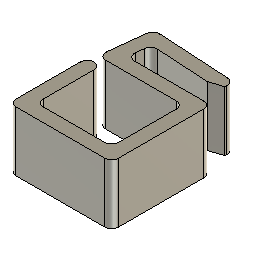
12 Gauge steel Wire Clip (Autodesk Fusion 360 design; units mm, degrees)
Autodesk Fusion 360 part; units mm, degrees
sketch "Sketch1" plane through (0, 0, 0) normal (0, 0, 1) x (1, 0, 0)
  line L0 (0, 0) -> (-9.9822, 0.5962)
  line L1 (-9.9822, 0.5962) -> (-10.6445, -5.2915)
  line L2 (-10.6445, -5.2915) -> (-0.6445, -5.2915)
  line L3 (-0.6445, -5.2915) -> (-0.6445, -13.6961)
  line L4 (-0.6445, -13.6961) -> (-9.4587, -13.6961)
  line L5 (-11.0587, -13.6961) -> (-11.0587, -15.2961)
  line L6 (-11.0587, -15.2961) -> (0.9555, -15.2961)
  line L7 (0.9555, -15.2961) -> (0.9555, -3.6915)
  line L8 (0.9555, -3.6915) -> (-8.8544, -3.6915)
  line L9 (-8.8544, -3.6915) -> (-8.562, -1.0915)
  line L10 (-8.562, -1.0915) -> (-0.0954, -1.5972)
  line L11 (-8.562, -1.0915) -> (-8.562, -3.6915) construction
  line L12 (0, 0) -> (-0.0954, -1.5972)
  line L13 (-11.0587, -13.6961) -> (-11.0587, -6.1692)
  line L14 (-11.0587, -6.1692) -> (-9.4587, -6.1692)
  line L15 (-9.4587, -6.1692) -> (-9.4587, -13.6961)
  dimension "d2" = 2.6
  dimension "d3" = 1.6
  dimension "d4" = 1.6
  dimension "d5" = 1.6
  dimension "d6" = 93
  dimension "d8" = 10
  dimension "d10" = 10
  dimension "d11" = 1.6
  dimension "d12" = 1.6
  dimension "d13" = 1.6
  constraint perpendicular L2 L3
  constraint perpendicular L3 L4
  constraint perpendicular L4 L5
  constraint perpendicular L5 L6
  constraint perpendicular L4 L7
  constraint perpendicular L7 L8
  constraint parallel L1 L9
  constraint parallel L0 L10
  constraint coincident L8 L11.end
  constraint perpendicular L8 L11
  constraint perpendicular L10 L12
  constraint coincident L0.start L12.start
  constraint perpendicular L4 L13
  constraint perpendicular L5 L14
  constraint perpendicular L4 L15
  measures "d2" distance of L9.end L11.end
  measures "d3" distance of L0 L10
  measures "d4" distance of L2 L8
  measures "d5" distance of L1 L9
  measures "d6" angle of L9 L10
  measures "d8" distance of L1.end L2.end
  measures "d10" distance of L0.start L0.end
  measures "d11" distance of L3 L7
  measures "d12" distance of L4 L6
  measures "d13" distance of L13 L15
extrude "Extrude1" add sketch "Sketch1" along normal blind 7
fillet "Fillet1" radius 0.8 13 edges at (-8.8544, -3.6915, 3.5) (-8.562, -1.0915, 3.5) (-9.4587, -13.6961, 3.5) (-0.6445, -5.2915, 3.5) (-0.6445, -13.6961, 3.5) (-9.9822, 0.5962, 3.5) (-10.6445, -5.2915, 3.5) (-11.0587, -6.1692, 3.5) (-9.4587, -6.1692, 3.5) (-11.0587, -15.2961, 3.5) (0.9555, -15.2961, 3.5) (0.9555, -3.6915, 3.5) (0, 0, 3.5)
chamfer "Chamfer1" distance 1.5 distance2 0.6 1 edges at (-0.0954, -1.5972, 3.5) measured on face at (-5.2347, -1.2902, 2.3333)
